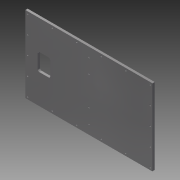
# Autodesk Inventor part: board
Saved by Autodesk Inventor 2015 (Build 190159000, 159)
## iProperties
Created: 2015-12-24
Part Number: board
Material: ステンレス鋼
Document SubType Name: Modeling
Designer: Ryo
Density: 8 g/cm^3
Appearance: 半つや出し
Author: Ryo
Autodesk Inventor part; units mm, degrees
ref_plane "YZ Plane" through (0, 0, 0) normal (1, 0, 0) x (0, 1, 0)
ref_plane "XZ Plane" through (0, 0, 0) normal (0, 1, 0) x (-1, 0, 0)
ref_plane "XY Plane" through (0, 0, 0) normal (0, 0, 1) x (1, 0, 0)
sketch "スケッチ1" plane through (0, 0, 0) normal (0, 1, 0) x (-1, 0, 0)
  line L0 (-550, 330) -> (550, 330)
  line L1 (550, 330) -> (550, -330)
  line L2 (550, -330) -> (-550, -330)
  line L3 (-550, -330) -> (-550, 330)
  line L4 (-550, 330) -> (550, -330) construction
  line L5 (550, 330) -> (-550, -330) construction
  line L6 (427, 75) -> (349, 75)
  line L7 (334, 60) -> (334, -60)
  line L8 (349, -75) -> (427, -75)
  line L9 (442, -60) -> (442, 60)
  line L10 (442, 75) -> (334, -75) construction
  line L11 (334, 75) -> (442, -75) construction
  arc A0 (442, 60) -> (427, 75) centre (427, 60) ccw
  arc A1 (349, 75) -> (334, 60) centre (349, 60) ccw
  arc A2 (427, -75) -> (442, -60) centre (427, -60) ccw
  arc A3 (334, -60) -> (349, -75) centre (349, -60) ccw
  circle A4 centre (-530, 310) radius 5
  circle A5 centre (-530, -310) radius 5
  circle A6 centre (-530, 0) radius 5
  circle A7 centre (-530, 155) radius 5
  circle A8 centre (-530, -155) radius 5
  line L12 (0, -462) -> (0, 462) projected
  circle A9 centre (530, 310) radius 5
  circle A10 centre (530, -310) radius 5
  circle A11 centre (530, 0) radius 5
  circle A12 centre (530, 155) radius 5
  circle A13 centre (530, -155) radius 5
  circle A14 centre (318, 310) radius 5
  circle A15 centre (106, 310) radius 5
  circle A16 centre (-106, 310) radius 5
  circle A17 centre (-318, 310) radius 5
  line L13 (770, 0) -> (-770, 0) projected
  circle A18 centre (318, -310) radius 5
  circle A19 centre (106, -310) radius 5
  circle A20 centre (-106, -310) radius 5
  circle A21 centre (-318, -310) radius 5
  point P0 (0, 0)
  point P1 (388, 0)
  point P2 (0, -250)
  point P3 (0, -125)
  point P4 (0, 125)
  point P5 (0, 250)
  dimension "d0" = 1100
  dimension "d1" = 660
  dimension "d2" = 108
  dimension "d3" = 108
  dimension "d4" = 150
  dimension "d5" = 255
  dimension "d6" = 15
  dimension "d7" = 15
  dimension "d8" = 10
  dimension "d9" = 20
  dimension "d10" = 20
  dimension "d11" = 10
  dimension "d12" = 20
  dimension "d13" = 20
  dimension "d14" = 10
  dimension "d15" = 10
  dimension "d16" = 155
  dimension "d17" = 10
  dimension "d18" = 155
  dimension "d19" = 20
  dimension "d20" = 20
  dimension "d21" = 20
  dimension "d24" = 212
  dimension "d185" = 80
  dimension "d186" = 205
  dimension "d187" = 80
  dimension "d188" = 205
  constraints: 24 end point, 22 centre point, 12 point on line, 9 symmetric about line, 8 point on circle, 8 tangent, 4 midpoint, 4 parallel, 3 horizontal, 2 equal radius, 2 perpendicular, 17 other
  measures "d0" distance of L1.end L2.end
  measures "d1" distance between parallel lines of L2 L0
  measures "d2" distance between parallel lines of L9 L1
  measures "d3" distance between parallel lines of L7 L9
  measures "d4" distance between parallel lines of L8 L6
  measures "d5" distance between parallel lines of L0 L6
  measures "d6" radius of A0
  measures "d7" radius of A1
  measures "d8" diameter of A4
  measures "d9" distance from line of L0 A4.centre
  measures "d10" distance from line of L3 A4.centre
  measures "d11" diameter of A5
  measures "d12" distance from line of L3 A5.centre
  measures "d13" distance from line of L2 A5.centre
  measures "d14" diameter of A6
  measures "d15" diameter of A7
  measures "d16" distance of A4.centre A7.centre
  measures "d17" diameter of A8
  measures "d18" distance of A5.centre A8.centre
  measures "d19" distance from line of L3 A8.centre
  measures "d20" distance from line of L3 A6.centre
  measures "d21" distance from line of L3 A7.centre
  measures "d24" distance of A9.centre A14.centre
  measures "d185" distance from line of point (0, -250) L2
  measures "d186" distance from line of L2 point (0, -125)
  measures "d187" distance from line of L0 point (0, 250)
  measures "d188" distance from line of point (0, 125) L0
extrude "押し出し1" add sketch "スケッチ1" along normal blind 20 contours L0 L12 L13 A6 L3 | L0 L1 L13 A11 L9 A0 L6 A1 L7 L12 | L13 A6 L12 L2 L3 | L13 L7 A3 L8 A2 L9 A11 L1 L2 L12
extrude "押し出し2" add sketch "スケッチ1" along normal blind 20 contours A9 | A14 | A15 | A16 | A17
extrude "押し出し3" cut sketch "スケッチ1" along normal blind 20 contours L13 A6 | A6 L13 | L13 A11 | A11 L13 | A4 | A5 | A7 | A8 | A10 | A12 | A13 | A17 | A18 | A19 | A20 | A21
extrude "押し出し4" add sketch "スケッチ1" along normal blind 20 contours L13 A11 | A11 L13 | A10 | A12 | A13 | A18 | A19
extrude "押し出し5" add sketch "スケッチ1" along normal blind 20 contours L0 L12 L13 A6 L3 | L0 L1 L13 A11 L9 A0 L6 A1 L7 L12 | L13 A6 L12 L2 L3 | L13 L7 A3 L8 A2 L9 A11 L1 L2 L12 | L13 A6 | A6 L13 | A5 | A8 | A20 | A21
extrude "押し出し6" add sketch "スケッチ1" along normal blind 20 contours L0 L12 L13 A6 L3 | L0 L1 L13 A11 L9 A0 L6 A1 L7 L12 | L13 A6 L12 L2 L3 | L13 L7 A3 L8 A2 L9 A11 L1 L2 L12 | A4 | A7 | A17
hole "穴1" at (530, 0, 310) direction (0, 1, 0) diameter 8 depth 20 counterbore diameter 12 counterbore depth 6
hole "穴2" at (318, 0, 310) direction (0, 1, 0) diameter 8 depth 20 counterbore diameter 12 counterbore depth 6
hole "穴3" at (106, 0, 310) direction (0, 1, 0) diameter 8 depth 20 counterbore diameter 12 counterbore depth 6
hole "穴4" at (-106, 0, 310) direction (0, 1, 0) diameter 8 depth 20 counterbore diameter 12 counterbore depth 6
hole "穴5" at (-318, 0, 310) direction (0, 1, 0) diameter 8 depth 20 counterbore diameter 12 counterbore depth 6
hole "穴6" at (-530, 0, 310) direction (0, 1, 0) diameter 8 depth 20 counterbore diameter 12 counterbore depth 6
hole "穴7" at (-530, 0, 155) direction (0, 1, 0) diameter 8 depth 20 counterbore diameter 12 counterbore depth 6
hole "穴8" at (-530, 0, 0) direction (0, 1, 0) diameter 8 depth 20 counterbore diameter 12 counterbore depth 6
hole "穴9" at (-530, 0, -155) direction (0, 1, 0) diameter 8 depth 20 counterbore diameter 12 counterbore depth 6
hole "穴10" at (-530, 0, -310) direction (0, 1, 0) diameter 8 depth 20 counterbore diameter 12 counterbore depth 6
hole "穴11" at (-318, 0, -310) direction (0, 1, 0) diameter 8 depth 20 counterbore diameter 12 counterbore depth 6
hole "穴12" at (-106, 0, -310) direction (0, 1, 0) diameter 8 depth 20 counterbore diameter 12 counterbore depth 6
hole "穴13" at (106, 0, -310) direction (0, 1, 0) diameter 8 depth 20 counterbore diameter 12 counterbore depth 6
hole "穴14" at (318, 0, -310) direction (0, 1, 0) diameter 8 depth 20 counterbore diameter 12 counterbore depth 6
hole "穴15" at (530, 0, -310) direction (0, 1, 0) diameter 8 depth 20 counterbore diameter 12 counterbore depth 6
hole "穴16" at (530, 0, -155) direction (0, 1, 0) diameter 8 depth 20 counterbore diameter 12 counterbore depth 6
hole "穴17" at (530, 0, 0) direction (0, 1, 0) diameter 8 depth 20 counterbore diameter 12 counterbore depth 6
hole "穴18" at (530, 0, 155) direction (0, 1, 0) diameter 8 depth 20 counterbore diameter 12 counterbore depth 6
fillet "フィレット1" radius 2 4 edges at (550, 10, -330) (-550, 10, -330) (-550, 10, 330) (550, 10, 330)
hole "穴19" at (0, 0, -250) at (0, 0, -125) at (0, 0, 125) at (0, 0, 250) direction (0, 1, 0) diameter 8 depth 20 counterbore diameter 12 counterbore depth 6
